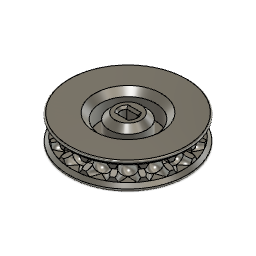
ball chain pulley v7 (Autodesk Fusion 360 design; units mm, degrees)
Autodesk Fusion 360 part; units mm, degrees
sketch "ball" plane through (0, 0, 0) normal (0, 1, 0) x (1, 0, 0)
  line L0 (0, 0) -> (64.6253, 0) construction
  circle A0 centre (16.9346, 0) radius 2.7
  line L1 (14.2346, 0) -> (19.6346, 0)
  line L2 (16.0111, -2.5372) -> (31.3304, -2.5372) construction
  line L3 (30.9346, -4.0506) -> (30.9346, 0)
  line L4 (30.9346, 0) -> (19.6346, 0)
  circle A1 centre (15.6455, -6.4806) radius 2.7
  circle A2 centre (0, 0) radius 16.9346 construction
  line L5 (19.0842, -4.5605) -> (31.0842, -4.5605) construction
  line L6 (16.9346, 0) -> (16.9346, -15.665) construction
  line L7 (0, 0) -> (37.1157, -15.3738) construction
  arc A3 (19.9854, -3.9637) -> (16.9346, -2.7) centre (16.9346, -7.0145) ccw
  line L8 (16.9346, -7.0145) -> (19.9854, -3.9637) construction
  line L9 (16.9346, -7.0145) -> (16.9346, -2.7) construction
  line L10 (30.9346, -4.0506) -> (30.9346, -29.2235)
  line L11 (19.9854, -3.9637) -> (31.7089, -15.6872)
  line L12 (19.9854, -3.9637) -> (36.565, -3.9637) construction
  point P0 (16.7193, -2.6914)
  point P1 (16.9346, -7.0145)
  point P2 (16.9346, -2.7)
  dimension "d10" = 5.4
  dimension "d11" = 16.9346
  dimension "d22" = 15
  dimension "d50" = -22.5
  dimension "d56" = 45
  dimension "d57" = 45
  dimension "d58" = 14
  constraint coincident L0.start A2.centre
  constraint horizontal L0
  constraint coincident L0 A0.centre
  constraint coincident A0 L1.start
  constraint coincident L0 L1.start
  constraint coincident A0 L1.end
  constraint coincident L0 L1.end
  constraint horizontal L2
  constraint coincident A0 L2.start
  constraint coincident L0 L3.end
  constraint perpendicular L0 L3
  constraint coincident A0.centre A2
  constraint coincident A0 P0
  constraint coincident A2 P0
  constraint horizontal L5
  constraint coincident A0.centre L6.start
  constraint tangent A2 L6
  constraint perpendicular L1 L6
  constraint coincident A1.centre L7
  constraint coincident L7 P1
  constraint coincident L6 P1
  constraint coincident A0 P2
  constraint coincident L6 P2
  constraint coincident P2 A3.end
  constraint coincident P1 A3.centre
  constraint perpendicular L4 L10
  constraint horizontal L12
  measures "d10" diameter of A0
  measures "d11" distance of L0.start A0.centre
  measures "d22" distance of L2.start L3.start
  measures "d56" angle of L8 L9
  measures "d57" angle of L11 L12
  measures "d58" distance of A0.centre L3
revolve "Revolve1" add sketch "ball" angle 360 about axis through (0, 0, 0) along (1, 0, 0) contours A0 L3 L4 A3 L10 L11 | A0 L1 picked at (16.1775, -0.7427) makes body 1
ref_plane "WorkPlane1" through (0, 2.7, 0) normal (0, 1, 0) x (0, 0, 1)
split "Split1" by plane through (0, 2.7, 0) normal (0, 1, 0) bodies 1 makes body 2 at (28.5014, 7.1081, -10.2576)
ref_plane "WorkPlane2" through (0, -2.7, 0) normal (0, 1, 0) x (0, 0, 1)
split "Split2" by plane through (0, -2.7, 0) normal (0, 1, 0) bodies 1 makes body 3 at (24.5355, 2.7, -1.0065)
delete_body "RemoveBody1" bodies 2
delete_body "RemoveBody2" bodies 1
pattern_circular "C-Pattern1" count 16 over 360 about axis through (0, 1.75, 0) along (0, 1, 0) of bodies 3 makes body 4 at (23.053, 2.7, -8.4594) makes body 5 at (18.0609, 2.7, -16.6375) makes body 6 at (10.3192, 2.7, -22.2826) makes body 7 at (-1.0065, 2.7, -24.5355) makes body 8 at (-10.3192, 2.7, -22.2826) makes body 9 at (-16.6375, 2.7, -18.0609) makes body 10 at (-23.053, 2.7, -8.4594) makes body 11 at (-24.5355, 2.7, 1.0065) makes body 12 at (-23.053, 2.7, 8.4594) makes body 13 at (-16.6375, 2.7, 18.0609) makes body 14 at (-10.3192, 2.7, 22.2826) makes body 15 at (1.0065, 2.7, 24.5355) makes body 16 at (10.3192, 2.7, 22.2826) makes body 17 at (16.6375, 2.7, 18.0609) makes body 18 at (22.2826, 2.7, 10.3192)
sketch "wire" plane through (0, 0, 0) normal (0, 0, 1) x (1, 0, 0)
  line L0 (0, 0) -> (20.6888, 0) construction
  circle A0 centre (16.9346, 0) radius 0.8
  line L1 (16.7957, 0.7878) -> (26.6437, 2.5243)
  line L2 (16.7957, 0.7878) -> (26.8362, 0.7878) construction
  line L3 (16.7957, -0.7878) -> (26.6437, -2.5243)
  line L4 (26.6437, 2.5243) -> (26.6437, -2.5243)
  dimension "d15" = 1.6
  dimension "d16" = 16.9346
  dimension "d17" = 10
  dimension "d18" = 10
  constraint coincident L0.start origin
  constraint horizontal L0
  constraint coincident L0 A0.centre
  constraint horizontal L2
  constraint coincident A0 L1.start
  constraint tangent A0 L1
  constraint symmetric L0 L1.start L3.start
  constraint symmetric L0 L1.end L3.end
  measures "d15" diameter of A0
  measures "d16" distance of L0.start A0.centre
  measures "d17" angle of L1 L2
  measures "d18" distance of L1.start L1.end
revolve "Revolve2" add sketch "wire" angle 360 about axis through (0, 1.75, 0) along (0, 1, 0) bodies 3 4 5 6 7 8 9 10 11 12 13 14 15 16 17 18
sketch "hub" plane through (0, 0, 0) normal (0, 1, 0) x (1, 0, 0)
  circle A0 centre (0, 0) radius 19.6346
  circle A1 centre (0, 0) radius 44.6346
  circle A2 centre (0, 0) radius 2.56
  line L0 (2.56, -1.58) -> (-2.56, -1.58)
  line L1 (-2.56, -1.58) -> (-2.56, 1.58)
  line L2 (-2.56, 1.58) -> (2.56, 1.58)
  line L3 (2.56, 1.58) -> (2.56, -1.58)
  line L4 (2.56, -1.58) -> (-2.56, 1.58) construction
  line L5 (-2.56, -1.58) -> (2.56, 1.58) construction
  circle A3 centre (0, 0) radius 6.56
  circle A4 centre (0, 0) radius 9.6346
  dimension "d26" = 39.2692
  dimension "d27" = 89.2692
  dimension "d30" = 5.12
  dimension "d40" = 5.12
  dimension "d41" = 3.16
  dimension "d42" = 13.12
  dimension "d43" = 19.2692
  constraint coincident A0.centre A1.centre
  constraint concentric A0 A1
  constraint horizontal L0
  constraint perpendicular L0 L1
  constraint parallel L0 L2
  constraint parallel L1 L3
  constraint coincident L4 A0.centre
  constraint coincident L5 A0.centre
  constraint concentric A2 A3
  constraint concentric A1 A4
  measures "d26" diameter of A0
  measures "d27" diameter of A1
  measures "d30" diameter of A2
  measures "d40" distance of L1.end L2.end
  measures "d41" distance of L0.end L1.end
  measures "d42" diameter of A3
  measures "d43" diameter of A4
extrude "Extrude1" cut sketch "hub" along normal mid plane 100 contours A1 bodies 3
extrude "Extrude2" add sketch "hub" along normal mid plane 9.4 separate body contours A0 | A2 L0 L3 | A2 L2 L3 | A2 L2 | A2 L0 | A2 L1 L2 | A2 L0 L1 | A3 | A4 makes body 19
combine "Combine1" operation cut target body 19 tool bodies 3
sketch "rim" plane through (0, 0, 0) normal (0, 0, 1) x (1, 0, 0)
  line L0 (19.4997, -2.7) -> (19.6346, -2.7)
  line L1 (-19.6346, -2.7) -> (-19.4997, -2.7)
  line L2 (19.6346, 2.7) -> (19.4997, 2.7)
  line L3 (-19.4997, 2.7) -> (-19.6346, 2.7)
  line L4 (19.6346, 4.7) -> (-19.6346, 4.7)
  line L5 (-19.6346, -4.7) -> (19.6346, -4.7)
  line L6 (19.6346, 2.7) -> (19.6346, 4.7)
  line L7 (-19.6346, 2.7) -> (-19.6346, 4.7)
  line L8 (19.6346, -4.7) -> (19.6346, -2.7)
  line L9 (-19.6346, -4.7) -> (-19.6346, -2.7)
  line L10 (19.6346, 2.7) -> (21.6346, 4.7)
  line L11 (19.6346, 2.7) -> (38.1243, 2.7) construction
  line L12 (21.6346, 4.7) -> (19.6346, 4.7)
  line L13 (20, 0) -> (2.5, 0)
  line L14 (21.6346, -4.7) -> (19.6346, -4.7)
  line L15 (19.6346, -2.7) -> (21.6346, -4.7)
  spline S0 degree 3 poles (-16.5993, -0.7878) (-16.5405, -0.7775) (-16.4824, -0.76) (-16.3406, -0.7012) (-16.2421, -0.6353) (-16.1025, -0.4956) (-16.0368, -0.3971) (-15.9613, -0.2147) (-15.9382, -0.0986) (-15.9382, 0.0986) (-15.9613, 0.2147) (-16.0368, 0.3971) (-16.1025, 0.4956) (-16.2421, 0.6353) (-16.3406, 0.7012) (-16.4824, 0.76) (-16.5405, 0.7775) (-16.5993, 0.7878) knots 0.131895 0.131895 0.131895 0.131895 0.14838 0.14838 0.178071 0.178071 0.207708 0.207708 0.237299 0.237299 0.26689 0.26689 0.296527 0.296527 0.326218 0.326218 0.342704 0.342704 0.342704 0.342704
  spline S1 degree 3 poles (16.5993, 0.7878) (16.5405, 0.7775) (16.4824, 0.76) (16.3406, 0.7012) (16.2421, 0.6353) (16.1025, 0.4956) (16.0368, 0.3971) (15.9613, 0.2147) (15.9382, 0.0986) (15.9382, -0.0986) (15.9613, -0.2147) (16.0368, -0.3971) (16.1025, -0.4956) (16.2421, -0.6353) (16.3406, -0.7012) (16.4824, -0.76) (16.5405, -0.7775) (16.5993, -0.7878) knots 0.131895 0.131895 0.131895 0.131895 0.14838 0.14838 0.178071 0.178071 0.207708 0.207708 0.237299 0.237299 0.26689 0.26689 0.296527 0.296527 0.326218 0.326218 0.342704 0.342704 0.342704 0.342704
  spline S2 degree 3 poles (-16.5993, 0.7878) (-16.7091, 0.8072) (-16.8216, 0.8268) (-16.9346, 0.8464) knots 0.01937 0.01937 0.01937 0.01937 0.052084 0.052084 0.052084 0.052084
  spline S3 degree 3 poles (16.5993, -0.7878) (16.7091, -0.8072) (16.8216, -0.8268) (16.9346, -0.8464) knots 0.711893 0.711893 0.711893 0.711893 0.744608 0.744608 0.744608 0.744608
  spline S4 degree 3 poles (16.9346, 0.8464) (16.8216, 0.8268) (16.7092, 0.8072) (16.5993, 0.7878) knots 0.791687 0.791687 0.791687 0.791687 0.824401 0.824401 0.824401 0.824401
  spline S5 degree 3 poles (-16.9346, -0.8464) (-16.8216, -0.8268) (-16.7092, -0.8072) (-16.5993, -0.7878) knots 1.484211 1.484211 1.484211 1.484211 1.516925 1.516925 1.516925 1.516925
  spline S6 degree 3 poles (-19.3713, -1.2884) (-19.3542, -1.2851) (-19.337, -1.2818) (-19.079, -1.2322) (-18.823, -1.1842) (-18.0351, -1.0393) (-17.486, -0.9417) (-16.9346, -0.8464) knots -0.261328 -0.261328 -0.261328 -0.261328 -0.255109 -0.255109 -0.168411 -0.168411 -0.000267 -0.000267 -0.000267 -0.000267
  spline S7 degree 3 poles (16.9346, -0.8464) (17.229, -0.8973) (17.5243, -0.9491) (18.1075, -1.0532) (18.3923, -1.1048) (18.9144, -1.2013) (19.1501, -1.2458) (19.3713, -1.2884) knots -0.341384 -0.341384 -0.341384 -0.341384 -0.251723 -0.251723 -0.161961 -0.161961 -0.080943 -0.080943 -0.080943 -0.080943
  spline S8 degree 3 poles (19.3713, -1.2884) (19.3827, -1.4809) (19.3963, -1.6676) (19.4381, -2.1616) (19.4692, -2.45) (19.4997, -2.7) knots -0.170282 -0.170282 -0.170282 -0.170282 -0.108772 -0.108772 -0.00038 -0.00038 -0.00038 -0.00038
  spline S9 degree 3 poles (-16.9346, 0.8464) (-17.229, 0.8973) (-17.5243, 0.9491) (-18.1075, 1.0532) (-18.3923, 1.1048) (-18.9144, 1.2013) (-19.1501, 1.2458) (-19.3713, 1.2884) knots -0.341384 -0.341384 -0.341384 -0.341384 -0.251723 -0.251723 -0.161961 -0.161961 -0.080943 -0.080943 -0.080943 -0.080943
  spline S10 degree 3 poles (-19.3713, 1.2884) (-19.3827, 1.4809) (-19.3963, 1.6676) (-19.4381, 2.1616) (-19.4692, 2.45) (-19.4997, 2.7) knots -0.170282 -0.170282 -0.170282 -0.170282 -0.108772 -0.108772 -0.00038 -0.00038 -0.00038 -0.00038
  spline S11 degree 3 poles (19.3713, 1.2884) (19.3542, 1.2851) (19.337, 1.2818) (19.079, 1.2322) (18.823, 1.1842) (18.0351, 1.0393) (17.486, 0.9417) (16.9346, 0.8464) knots -0.261328 -0.261328 -0.261328 -0.261328 -0.255109 -0.255109 -0.168411 -0.168411 -0.000267 -0.000267 -0.000267 -0.000267
  spline S12 degree 3 poles (-19.4997, -2.7) (-19.4691, -2.4498) (-19.438, -2.1612) (-19.3963, -1.6671) (-19.3827, -1.4807) (-19.3713, -1.2884) knots -0.216275 -0.216275 -0.216275 -0.216275 -0.107685 -0.107685 -0.046191 -0.046191 -0.046191 -0.046191
  spline S13 degree 3 poles (19.4997, 2.7) (19.4691, 2.4498) (19.438, 2.1612) (19.3963, 1.6671) (19.3827, 1.4807) (19.3713, 1.2884) knots -0.216275 -0.216275 -0.216275 -0.216275 -0.107685 -0.107685 -0.046191 -0.046191 -0.046191 -0.046191
  dimension "d34" = 45
  constraint horizontal L11
  constraint coincident L2.start L6.start
  constraint coincident L4.start L6.end
  constraint perpendicular L6 L12
  constraint symmetric L2.start L13 L0.end
  constraint symmetric L10.end L13 L14.start
  constraint symmetric L4.start L13 L5.end
  measures "d34" angle of L10 L11
revolve "Revolve3" add sketch "rim" angle 360 about axis through (0, 1.75, 0) along (0, 1, 0) contours L8 L14 L15 | L6 L10 L12 bodies 19
fillet "Fillet1" radius 0.5 2 edges at (-20.1705, 4.7, -7.8234) (-20.1705, -4.7, -7.8234) on bodies 19
extrude "Extrude3" cut sketch "hub" against normal blind 7.4 from surface at 4.7 contours A4 bodies 19
chamfer "Chamfer1" distance 2 angle 45 2 edges at (-6.1161, 4.7, 2.3722) (-8.9826, 4.7, -3.484) on bodies 19
chamfer "Chamfer2" distance 0.75 angle 45 4 edges at (0, 4.7, -1.58) (-2.56, 4.7, 0) (0, 4.7, 1.58) (2.56, 4.7, 0) on bodies 19
equation "ballDia = _5mmBallDia"
equation "ballSpacing = _5mmBallSpacing"
equation "wireDia = 1.2 mm"
equation "numBalls = 16"
equation "pulleyCircumference = numBalls * ballSpacing"
equation "pulleyDia = pulleyCircumference / 3.1415"
equation "ballClearance = 0.2 mm"
equation "ballHoleDia = ballDia + 2 * ballClearance"
equation "d10 = ballHoleDia"
equation "d11 = pulleyDia / 2"
equation "d13 = numBalls"
equation "d15 = wireDia + 2 * ballClearance"
equation "d16 = pulleyDia / 2"
equation "coneAngle = 20 deg"
equation "d23 = ballHoleDia / 2"
equation "d24 = -ballHoleDia / 2"
equation "pulleyOuterDia = pulleyDia + ballHoleDia"
equation "d26 = pulleyOuterDia"
equation "d27 = pulleyOuterDia + 50 mm"
equation "d30 = spindleDia"
equation "pulleyThickness = ballHoleDia + 4 mm"
equation "d32 = pulleyThickness"
equation "spindleDia = 4.92 mm + 0.2 mm"
equation "spindleAF = 2.96 mm + 0.2 mm"
equation "d40 = spindleDia"
equation "d41 = spindleAF"
equation "d42 = spindleDia + 8 mm"
equation "d43 = pulleyOuterDia - 4 * ballDia"
equation "d45 = -( pulleyThickness - 2 mm )"
equation "d50 = ( -360 / numBalls ) * 1 deg"
equation "_5mmBallDia = 5 mm"
equation "_5mmBallSpacing = 6.65 mm"
named bodies: "pulley"
